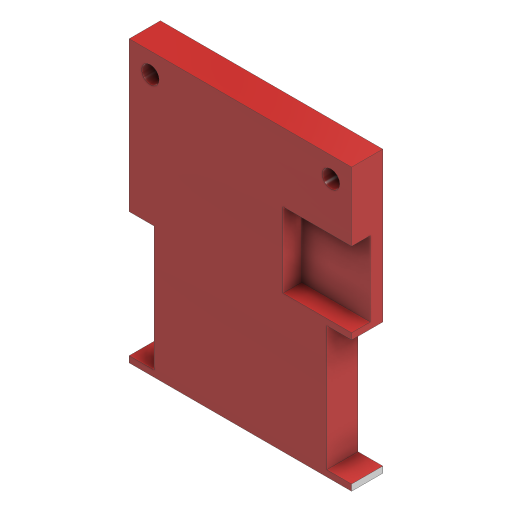
# Autodesk Inventor part: Качель камеры
Saved by Autodesk Inventor 2023.2 (Build 272271030, 271C)
## iProperties
Created: 2024-02-27
Part Number: Качель камеры
Material: Типовые
Document SubType Name: Modeling
Designer: liza
Density: 1 g/cm^3
Appearance: По умолчанию
Author: liza
Autodesk Inventor part; units mm, degrees
ref_plane "YZ Plane" through (0, 0, 0) normal (1, 0, 0) x (0, 1, 0)
ref_plane "XZ Plane" through (0, 0, 0) normal (0, 1, 0) x (-1, 0, 0)
ref_plane "XY Plane" through (0, 0, 0) normal (0, 0, 1) x (1, 0, 0)
sketch "Эскиз1" plane through (0, 0, 0) normal (0, 0, 1) x (1, 0, 0)
  line L0 (0, 0) -> (35.65, 0)
  line L1 (35.65, 0) -> (35.65, -45)
  line L2 (35.65, -45) -> (0, -45)
  line L3 (0, -45) -> (0, 0)
  dimension "d0" = 35.65
  dimension "d1" = 45
  constraints: 8 end point, 2 parallel, 1 horizontal, 1 perpendicular
  measures "d0" distance of L0.start L0.end
  measures "d1" distance of L0.end L1.end
extrude "Выдавливание1" add sketch "Эскиз1" along normal blind 5
sketch "Эскиз7" plane through (0, 0, 0) normal (0, 0, -1) x (-1, 0, 0)
  circle A0 centre (-32.35, -3.3) radius 1.4 projected
  circle A1 centre (-3.39, -3.3) radius 1.4 projected
  line L0 (-3.9799, -24) -> (1.0201, -24)
  line L1 (1.0201, -24) -> (1.0201, -44)
  line L2 (1.0201, -44) -> (-3.9799, -44)
  line L3 (-3.9799, -44) -> (-3.9799, -24)
  line L4 (0, -45) -> (-35.65, -45) construction
  line L5 (-17.825, -45) -> (-17.825, 0) construction
  line L6 (-35.65, 0) -> (0, 0) construction
  line L7 (-31.6701, -24) -> (-36.6701, -24)
  line L8 (-36.6701, -24) -> (-36.6701, -44)
  line L9 (-36.6701, -44) -> (-31.6701, -44)
  line L10 (-31.6701, -44) -> (-31.6701, -24)
  line L11 (0, 0) -> (0, -45) construction
  point P0 (0, -18.6108)
  dimension "d14" = 1
  dimension "d15" = 20
  dimension "d24" = 5
  constraints: 18 end point, 4 symmetric about line, 2 midpoint, 2 parallel, 1 horizontal, 1 perpendicular
  measures "d14" distance between parallel lines of L4 L2
  measures "d15" distance of L2.end L0.start
  measures "d24" distance of L0.start L0.end
extrude "Выдавливание3" cut sketch "Эскиз7" against normal through all
sketch "Эскиз9" plane through (0, 0, 5) normal (0, 0, 1) x (1, 0, 0)
  line L0 (35.65, -45) -> (35.65, 0) projected
  line L1 (35.65, -11) -> (24.65, -11)
  line L2 (24.65, -11) -> (24.65, -23)
  line L3 (24.65, -23) -> (35.65, -23)
  line L4 (35.65, -23) -> (35.65, -11)
  point P0 (0, 0)
  dimension "d19" = 11
  dimension "d20" = 12
  dimension "d21" = 11
  constraints: 8 end point, 2 parallel, 1 horizontal, 1 perpendicular, 1 point on line
  measures "d19" distance of L1.start L0.end
  measures "d20" distance of L1.end L2.end
  measures "d21" distance of L2.end L3.end
extrude "Выдавливание4" cut sketch "Эскиз9" against normal blind 3
